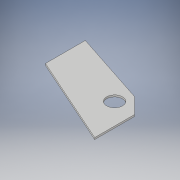
# Autodesk Inventor part: StorageGusset.ver1-1111-2020
Saved by Autodesk Inventor 2018 (Build 220112000, 112)
## iProperties
Created: 2020-01-27
Part Number: StorageGusset.ver1-1111-2020
Material: Generic
Document SubType Name: Modeling
Designer: Power Hawks CADD
Density: 1 g/cm^3
Appearance: Default
Author: Power Hawks CADD
Autodesk Inventor part; units mm, degrees
ref_plane "YZ Plane" through (0, 0, 0) normal (1, 0, 0) x (0, 1, 0)
ref_plane "XZ Plane" through (0, 0, 0) normal (0, 1, 0) x (-1, 0, 0)
ref_plane "XY Plane" through (0, 0, 0) normal (0, 0, 1) x (1, 0, 0)
sketch "Sketch1" plane through (0, 0, 0) normal (0, 1, 0) x (-1, 0, 0)
  line L0 (0, 0) -> (0, -71.8312)
  line L1 (0, 0) -> (159.893, -71.189)
  line L2 (159.893, -71.189) -> (159.893, -143.0202)
  line L3 (159.893, -143.0202) -> (0, -71.8312)
  circle A0 centre (96.393, -74.364) radius 14.2875
  line L4 (0, -71.8312) -> (27.94, -99.7712)
  line L5 (27.94, -99.7712) -> (159.893, -143.0202)
  point P0 (38.467, -74.3966)
  dimension "d0" = 71.8312
  dimension "d1" = 66
  dimension "d2" = 159.893
  dimension "d4" = 71.8312
  dimension "d5" = 3.175
  dimension "d6" = 63.5
  dimension "d7" = 28.575
  dimension "d10" = 38.467
  dimension "d11" = 74.3966
  dimension "d12" = 27.94
  dimension "d14" = 21
  constraints: 12 end point, 2 vertical, 1 centre point, 1 coincident
  measures "d0" distance of L0.start L0.end
  measures "d1" angle of L0 L1
  measures "d2" horizontal distance of L0.start L1.end
  measures "d4" distance of L1.end L2.end
  measures "d5" vertical distance of L1.end point (96.393, -74.364)
  measures "d6" distance from line of L2 point (96.393, -74.364)
  measures "d7" diameter of A0
  measures "d10" distance from line of point (38.467, -74.397) L0
  measures "d11" vertical distance of point (38.467, -74.397) L0.start
  measures "d12" distance from line of L0 L4.end
  measures "d14" angle of L3 L4
extrude "Extrusion1" add sketch "Sketch1" along normal blind 3.175 contours L1 L2 L3 L0
extrude "Extrusion2" add sketch "Sketch1" along normal blind 3.175 contours L3 L5 L4 | A0
hole "Hole1" at (-38.467, 0, -74.3966) direction (0, 1, 0) diameter 28.575 end through all
body "Solid1"
